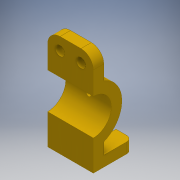
# Autodesk Inventor part: T05
Saved by Autodesk Inventor 2018 (Build 220112000, 112)
## iProperties
Created: 2020-06-26
Part Number: T05
Material: Generic
Document SubType Name: Modeling
Designer: Brandon Portillo
Density: 1 g/cm^3
Appearance: Gold
Author: Brandon Portillo
Autodesk Inventor part; units mm, degrees
ref_plane "YZ Plane" through (0, 0, 0) normal (1, 0, 0) x (0, 1, 0)
ref_plane "XZ Plane" through (0, 0, 0) normal (0, 1, 0) x (-1, 0, 0)
ref_plane "XY Plane" through (0, 0, 0) normal (0, 0, 1) x (1, 0, 0)
sketch "Sketch1" plane through (0, 0, 0) normal (1, 0, 0) x (0, 1, 0)
  line L0 (0, 0) -> (0, 32)
  arc A0 (0, 32) -> (0, 70) centre (0, 51) ccw
  line L1 (0, 70) -> (0, 107)
  line L2 (0, 0) -> (41, 0)
  line L3 (11, 107) -> (11, 78.9106)
  arc A1 (11, 23.0894) -> (11, 78.9106) centre (0, 51) ccw
  line L4 (11, 23.0894) -> (11, 11)
  line L5 (11, 11) -> (41, 11)
  line L6 (11, 107) -> (0, 107)
  line L7 (41, 11) -> (41, 0)
  dimension "d0" = 32
  dimension "d1" = 70
  dimension "d2" = 37
  dimension "d3" = 41
  dimension "d4" = 11
  constraints: 16 end point, 4 point on circle, 3 perpendicular, 2 centre point, 2 vertical, 1 horizontal, 1 point on line, 3 other
  measures "d0" distance of L0.start L0.end
  measures "d1" distance of L0.start L1.start
  measures "d2" distance of L1.start L1.end
  measures "d3" distance of L0.start L2.end
  measures "d4" distance between parallel lines of L0 L4
extrude "Extrusion1" add sketch "Sketch1" along normal blind 48
fillet "Fillet1" radius 13 1 edges at (48, 5.5, 107)
fillet "Fillet2" radius 13 1 edges at (0, 5.5, 107)
sketch "Sketch2" plane through (0, 11, 78.9106) normal (0, 1, 0) x (1, 0, 0)
  arc A0 (0, -15.0894) -> (13, -28.0894) centre (13, -15.0894) ccw projected
  circle A1 centre (13, -15.0894) radius 5
  arc A2 (35, -28.0894) -> (48, -15.0894) centre (35, -15.0894) ccw projected
  circle A3 centre (35, -15.0894) radius 5
  point P0 (0, 78.9106)
  dimension "d9" = 10
  dimension "d10" = 10
  constraints: 2 centre point, 2 coincident
  measures "d9" diameter of A1
  measures "d10" diameter of A3
extrude "Extrusion2" cut sketch "Sketch2" against normal blind 11
fillet "Fillet3" radius 6 1 edges at (48, 41, 5.5)
fillet "Fillet4" radius 6 1 edges at (0, 41, 5.5)
sketch "Sketch3" plane through (48, 0, 0) normal (0, 0, -1) x (-1, 0, 0)
  line L0 (57.6, 0) -> (-9.6, 0) construction
  line L1 (48, -8.2) -> (48, 49.2) projected
  arc A0 (17.1801, 25) -> (30.1801, 25) centre (23.6801, 25) ccw
  line L2 (17.1801, 25) -> (17.1801, 41)
  line L3 (42, 41) -> (6, 41) projected
  line L4 (30.1801, 25) -> (30.1801, 41)
  point P0 (48, 0)
  dimension "d15" = 25
  dimension "d16" = 13
  constraints: 4 end point, 2 point on circle, 2 point on line, 1 centre point, 1 coincident, 1 parallel, 1 vertical
  measures "d15" distance from line of L0 point (23.68, 25)
  measures "d16" diameter of A0
extrude "Extrusion3" cut sketch "Sketch3" against normal blind 11
sketch "Sketch4" plane through (0, 0, 0) normal (0, -1, 0) x (1, 0, 0)
  line L0 (0, 32) -> (48, 32) projected
  line L1 (0, 32) -> (0, 70) projected
  circle A0 centre (24, 51) radius 2.5
  point P0 (0, 0)
  point P1 (24, 32)
  point P2 (0, 51)
  dimension "d19" = 24
  dimension "d20" = 5
  constraints: 2 midpoint, 1 centre point, 1 coincident, 1 horizontal alignment
  measures "d19" distance of point (0, 51) point (24, 51)
  measures "d20" diameter of A0
extrude "Extrusion4" cut sketch "Sketch4" against normal blind 41
body "Solid1"
